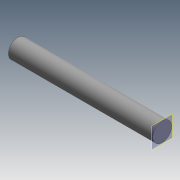
# Autodesk Inventor part: 6-32 Rod
Saved by Autodesk Inventor 2014 SP1 (Build 180222100, 222)
## iProperties
Created: 2014-04-09
Part Number: 6-32 Rod
Material: Generic
Document SubType Name: Modeling
Designer: tom
Density: 1 g/cm^3
Appearance: Default
Author: tom
Autodesk Inventor part; units mm, degrees
ref_plane "YZ Plane" through (0, 0, 0) normal (1, 0, 0) x (0, 1, 0)
ref_plane "XZ Plane" through (0, 0, 0) normal (0, 1, 0) x (-1, 0, 0)
ref_plane "XY Plane" through (0, 0, 0) normal (0, 0, 1) x (1, 0, 0)
ref_plane "Work Plane1" through (80.091, -13.6313, -17.8808) normal (-1, 0, 0) x (0, -1, 0)
sketch "Sketch1" plane through (80.091, -13.6313, -17.8808) normal (-1, 0, 0) x (0, -1, 0)
  circle A0 centre (0, 0) radius 1.65
  point P0 (-13.6313, 17.8808)
  constraints: 1 centre point
extrude "Extrusion1" add sketch "Sketch1" along normal blind 103.15
thread "Thread1" size "6-32 UNC" class "2A" standard "ANSI Unified Screw Threads" full length
body "Solid1"
